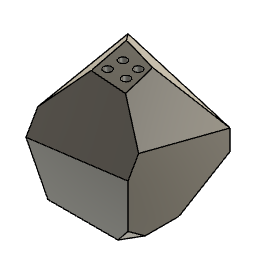
Suètone-drawing-object-03 v7 (Autodesk Fusion 360 design; units mm, degrees)
Autodesk Fusion 360 part; units mm, degrees
sketch "Esquisse1" plane through (0, 0, 0) normal (0, 0, 1) x (1, 0, 0)
  line L0 (50, 50) -> (-50, 50)
  line L1 (-50, 50) -> (-50, -50)
  line L2 (-50, -50) -> (50, -50)
  line L3 (50, -50) -> (50, 50)
  line L4 (50, 50) -> (-50, -50) construction
  line L5 (-50, 50) -> (50, -50) construction
  dimension "d1" = 100
  dimension "d2" = 100
  constraint horizontal L0
  constraint perpendicular L0 L1
  constraint parallel L0 L2
  constraint parallel L1 L3
  constraint coincident L4 origin
  constraint coincident L5 origin
  measures "d1" distance of L1.end L2.end
  measures "d2" distance of L0.end L1.end
extrude "Extrusion1" add sketch "Esquisse1" along normal blind 100 makes body 1
sketch "Esquisse2" plane through (0, 50, 0) normal (0, 1, 0) x (-1, 0, 0)
  line L0 (-50, 0) -> (50, 0)
  line L1 (50, 0) -> (50, 100)
  line L2 (50, 100) -> (-50, 100)
  line L3 (-50, 100) -> (-50, 0)
  line L4 (-50, 50) -> (50, 80)
  constraint midpoint L3 L4.start
  constraint coincident L1 L4.end
ref_plane "Plan de construction1" through (0, 50, 65) normal (0.203186, 0.707107, 0.677285) x (-0.957826, 0, 0.287348)
split "Scinder1" by plane through (0, 50, 65) normal (0.203186, 0.707107, 0.677285) bodies 1 makes body 2 at (16.6667, 50, 76.6667)
sketch "Esquisse3" plane through (50, 0, 0) normal (1, 0, 0) x (0, 1, 0)
  line L0 (50, 50) -> (2.1087, 100)
  line L1 (2.1087, 100) -> (-50, 100)
  line L2 (-50, 100) -> (-50, 0)
  line L3 (-50, 0) -> (50, 0)
  line L4 (50, 0) -> (50, 50)
  line L5 (-50, 75.825) -> (50, 50)
  constraint coincident L2 L5.start
  constraint coincident L0.start L4.end
ref_plane "Plan de construction2" through (50, 0, 62.9125) normal (0.707107, 0.176809, 0.684645) x (0, 0.968234, -0.250046)
split "Scinder2" by plane through (50, 0, 62.9125) normal (0.707107, 0.176809, 0.684645) bodies 1 makes body 3 at (50, 0.7029, 75.275)
sketch "Esquisse4" plane through (-50, 0, 0) normal (-1, 0, 0) x (0, -1, 0)
  line L0 (-30.8435, 100) -> (-50, 80)
  line L1 (-50, 80) -> (-50, 0)
  line L2 (-50, 0) -> (50, 0)
  line L3 (50, 0) -> (50, 100)
  line L4 (50, 100) -> (-30.8435, 100)
  line L5 (-50, 80) -> (50, 60)
  constraint coincident L0.end L1.start
  constraint coincident L3 L5.end
ref_plane "Plan de construction3" through (-50, 0, 70) normal (0.707107, 0.138675, -0.693375) x (0, -0.980581, -0.196116)
split "Scinder3" by plane through (-50, 0, 70) normal (0.707107, 0.138675, -0.693375) bodies 1 makes body 4 at (-16.6667, 16.6667, 0)
sketch "Esquisse5" plane through (0, -50, 0) normal (0, -1, 0) x (1, 0, 0)
  line L0 (-10.7768, 100) -> (-50, 60)
  line L1 (-50, 60) -> (-50, 0)
  line L2 (-50, 0) -> (50, 0)
  line L3 (50, 0) -> (50, 75.825)
  line L4 (50, 75.825) -> (26.5929, 100)
  line L5 (26.5929, 100) -> (-10.7768, 100)
  line L6 (-50, 42.1052) -> (50, 54.9508)
  constraint coincident L1 L6.start
  constraint coincident L3 L6.end
ref_plane "Plan de construction4" through (0, -50, 48.528) normal (0.063705, 0.866025, -0.495925) x (0.99185, 0, 0.12741)
split "Scinder4" by plane through (0, -50, 48.528) normal (0.063705, 0.866025, -0.495925) bodies 4 makes body 5 at (-16.6667, 16.6667, 0)
sketch "Esquisse6" plane through (50, 0, 0) normal (1, 0, 0) x (0, 1, 0)
  line L0 (-39.5865, 73.1357) -> (-50, 54.9508)
  line L1 (-50, 54.9508) -> (-50, 0)
  line L2 (-50, 0) -> (50, 0)
  line L3 (50, 0) -> (50, 50)
  line L4 (50, 50) -> (-39.5865, 73.1357)
  line L5 (0, 0) -> (50, 30)
  constraint coincident L5.start origin
  constraint coincident L3 L5.end
ref_plane "Plan de construction5" through (50, 25, 15) normal (0.707107, 0.363803, -0.606339) x (0, 0.857493, 0.514496)
split "Scinder5" by plane through (50, 25, 15) normal (0.707107, 0.363803, -0.606339) bodies 5 makes body 6 at (50, 33.3333, 10)
sketch "Esquisse7" plane through (0, 0, 100) normal (0, 0, 1) x (-1, 0, 0)
  line L0 (16.7997, 19.289) -> (-19.583, 21.9653)
  line L1 (-19.583, 21.9653) -> (-10.7427, -13.3892)
  line L2 (-10.7427, -13.3892) -> (25.2359, -23.7276)
  line L3 (25.2359, -23.7276) -> (16.7997, 19.289)
  circle A0 centre (10, 10) radius 4
  circle A1 centre (-7.059, 8.9606) radius 4
  circle A2 centre (10, -5) radius 4
  circle A3 centre (-5, -5) radius 4
  dimension "d10" = 8
  dimension "d11" = 8
  dimension "d12" = 8
  dimension "d13" = 8
  measures "d10" diameter of A0
  measures "d11" diameter of A1
  measures "d12" diameter of A2
  measures "d13" diameter of A3
extrude "Extrusion2" cut sketch "Esquisse7" against normal blind 175 contours A0 | A1 | A2 | A3 bodies 5
sketch "Esquisse8" plane through (-50, 0, 0) normal (-1, 0, 0) x (0, -1, 0)
  line L0 (50, 42.1052) -> (38.4272, 62.3146)
  line L1 (38.4272, 62.3146) -> (-50, 80)
  line L2 (-50, 80) -> (-50, 0)
  line L3 (-50, 0) -> (50, 0)
  line L4 (50, 0) -> (50, 42.1052)
  line L5 (-50, 40) -> (0, 0)
  constraint midpoint L2 L5.start
  constraint coincident L5.end origin
ref_plane "Plan de construction6" through (-50, 25, 20) normal (0.707107, -0.441726, 0.552158) x (0, -0.780869, -0.624695)
split "Scinder6" by plane through (-50, 25, 20) normal (0.707107, -0.441726, 0.552158) bodies 5 makes body 7 at (-3.0366, -37.9666, 0)
sketch "Esquisse9" plane through (50, 0, 0) normal (1, 0, 0) x (0, 1, 0)
  line L0 (0, 0) -> (50, 30)
  line L1 (50, 30) -> (50, 50)
  line L2 (50, 50) -> (-39.5865, 73.1357)
  line L3 (-39.5865, 73.1357) -> (-50, 54.9508)
  line L4 (-50, 54.9508) -> (-50, 0)
  line L5 (-50, 0) -> (0, 0)
  line L6 (-50, 12.1189) -> (-33.1708, 0)
  constraint coincident L4 L6.start
  constraint coincident L5 L6.end
ref_plane "Plan de construction7" through (50, -41.5854, 6.0595) normal (0.707107, -0.413208, -0.573811) x (0, 0.811491, -0.584365)
split "Scinder7" by plane through (50, -41.5854, 6.0595) normal (0.707107, -0.413208, -0.573811) bodies 7 makes body 8 at (50, -44.3903, 4.0396)
sketch "Esquisse10" plane through (-50, 0, 0) normal (-1, 0, 0) x (0, -1, 0)
  line L0 (-50, 40) -> (0, 0)
  line L1 (0, 0) -> (50, 0)
  line L2 (50, 0) -> (50, 42.1052)
  line L3 (50, 42.1052) -> (38.4272, 62.3146)
  line L4 (38.4272, 62.3146) -> (-50, 80)
  line L5 (-50, 80) -> (-50, 40)
  line L6 (50, 42.1052) -> (25, 0)
  constraint coincident L2.end L3.start
  constraint midpoint L1 L6.end
ref_plane "Plan de construction8" through (-50, -37.5, 21.0526) normal (0.707107, 0.608009, 0.361006) x (0, 0.51054, -0.859854)
split "Scinder8" by plane through (-50, -37.5, 21.0526) normal (0.707107, 0.608009, 0.361006) bodies 7 makes body 9 at (6.1407, -37.6498, 0)
hidden bodies 1 2 3 4 5 6 7 8
